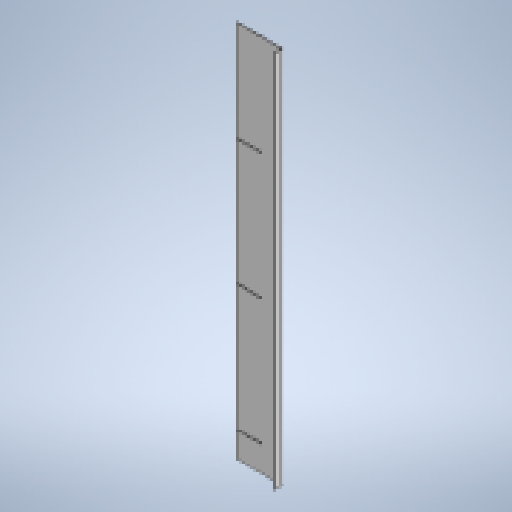
# Autodesk Inventor part: stringer 1.2
Saved by Autodesk Inventor 2026.2 (Build 302298000, 298)
## iProperties
Created: 2026-05-07
Part Number: stringer 1.2
Material: Steel
Document SubType Name: Sheet Metal
Designer: admin
Density: 7.85 g/cm^3
Sheet Metal Rule: Default_mm
Appearance: Default
Author: admin
Autodesk Inventor part; units mm, degrees
ref_plane "YZ Plane" through (0, 0, 0) normal (1, 0, 0) x (0, 1, 0)
ref_plane "XZ Plane" through (0, 0, 0) normal (0, 1, 0) x (-1, 0, 0)
ref_plane "XY Plane" through (0, 0, 0) normal (0, 0, 1) x (1, 0, 0)
sketch "Sketch1" plane through (0, 0, 0) normal (0, 0, 1) x (1, 0, 0)
  line L0 (0, 0) -> (-179.6388, 0)
  line L1 (-179.6388, 0) -> (-179.6388, -1500)
  line L2 (-179.6388, -1500) -> (0, -1500)
  line L3 (0, -1500) -> (0, 0)
  line L4 (-179.6388, -1400) -> (-81, -1400)
  line L5 (-81, -1400) -> (-81, -1394)
  line L6 (-81, -1394) -> (-179.6388, -1394)
  line L7 (-179.6388, -1394) -> (-179.6388, -1400)
  line L8 (-179.6388, -900) -> (-81, -900)
  line L9 (-81, -900) -> (-81, -894)
  line L10 (-81, -894) -> (-179.6388, -894)
  line L11 (-179.6388, -894) -> (-179.6388, -900)
  line L12 (-179.6388, -400) -> (-81, -400)
  line L13 (-81, -400) -> (-81, -394)
  line L14 (-81, -394) -> (-179.6388, -394)
  line L15 (-179.6388, -394) -> (-179.6388, -400)
  point P0 (-179.6388, -394)
  point P1 (-179.6388, -400)
  point P2 (-179.6388, -1394)
  dimension "d0" = 1500
  dimension "d1" = 179.6388
  dimension "d2" = 6
  dimension "d4" = 100
  dimension "d7" = 500
  dimension "d23" = 81
  measures "d0" distance of L1.end L0.end
  measures "d1" distance of L1.end L2.end
  measures "d2" distance of L4.end L5.end
  measures "d4" distance between parallel lines of L2 L4
  measures "d7" distance of L4.start L8.start
  measures "d23" distance between parallel lines of L3 L5
extrude "Plate1" add sketch "Sketch1" along normal blind 4 contours L3 L2 L1 L4 L5 L6 L8 L9 L10 L12 L13 L14 L0
sketch "Sketch2" plane through (4, 0, 0) normal (-1, 0, 0) x (0, -1, 0)
  line L0 (1500, 0) -> (0, 0)
  line L1 (0, 0) -> (0, 35)
  line L2 (0, 35) -> (1500, 35)
  line L3 (1500, 35) -> (1500, 0)
  constraints: 6 end point, 1 horizontal, 1 perpendicular, 1 vertical
edge flange "Flange1" height 35 angle 90 thickness 4 bend radius 4 thickness toward (-1, 0, 0) relief tear relief width 4 relief depth 2 edges at (0, -750, 4) wall of the first edge with corners at (4, -1500, 0) (4, 0, 0) (4, 0, 35) (4, -1500, 35)
bend "Bend1"
corner "Corner1"
equation "\"d1\" = Stringer2_deep"
equation "\"d12\" = Thickness"
equation "\"d13\" = BendReliefWidth"
equation "\"d14\" = BendReliefDepth"
equation "\"d15\" = MinimumRemnant"
equation "\"d16\" = TransitionRadius"
equation "\"d19\" = BendRadius"
equation "\"d20\" = CornerReliefSize"
equation "\"d21\" = GapSize"
equation "\"d22\" = JacobiRadiusSize"
equation "\"BendRadius\" = Thickness"
equation "\"BendReliefWidth\" = Thickness"
equation "\"BendReliefDepth\" = 0.5 * Thickness"
equation "\"CornerReliefSize\" = 4 * Thickness"
equation "\"MinimumRemnant\" = 2 * Thickness"
equation "\"TransitionRadius\" = BendRadius"
equation "\"JacobiRadiusSize\" = BendRadius"
equation "\"GapSize\" = Thickness"
equation "\"Stringer2_deep\" = 179.638781"
equation "\"Thickness\" = 4"
body "Solid1"
